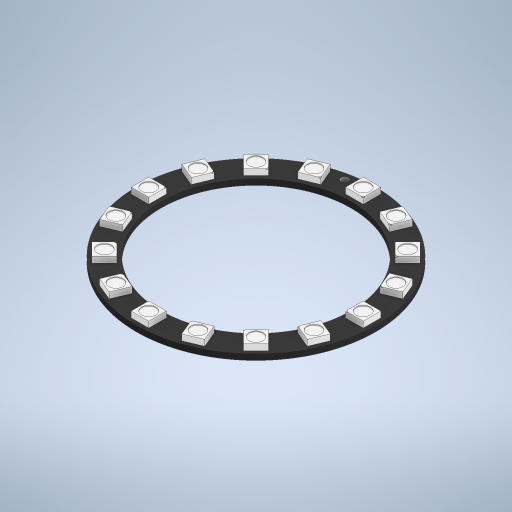
# Autodesk Inventor part: Neopixel circle
Saved by Autodesk Inventor 2023 (Build 270158000, 158)
## iProperties
Created: 2022-05-23
Part Number: Neopixel circle
Material: 일반
Document SubType Name: Modeling
Designer: user
Density: 1 g/cm^3
Appearance: 기본값
Author: user
Autodesk Inventor part; units mm, degrees
ref_plane "YZ Plane" through (0, 0, 0) normal (1, 0, 0) x (0, 1, 0)
ref_plane "XZ Plane" through (0, 0, 0) normal (0, 1, 0) x (-1, 0, 0)
ref_plane "XY Plane" through (0, 0, 0) normal (0, 0, 1) x (1, 0, 0)
sketch "스케치2" plane through (0, 0, 0) normal (0, 1, 0) x (-1, 0, 0)
  circle A0 centre (0, 0) radius 34
  circle A1 centre (0, 0) radius 27
  line L0 (33, 2.5) -> (28, 2.5)
  line L1 (28, 2.5) -> (28, -2.5)
  line L2 (28, -2.5) -> (33, -2.5)
  line L3 (33, -2.5) -> (33, 2.5)
  line L4 (33, 2.5) -> (28, -2.5) construction
  line L5 (28, 2.5) -> (33, -2.5) construction
  point P0 (30.5, 0)
  dimension "d0" = 68
  dimension "d1" = 54
  dimension "d2" = 5
  dimension "d3" = 5
  dimension "d4" = 33
  constraints: 12 end point, 2 centre point, 2 coincident, 2 midpoint, 2 parallel, 1 horizontal, 1 perpendicular
  measures "d0" diameter of A0
  measures "d1" diameter of A1
  measures "d2" distance of L2.end L1.end
  measures "d3" distance of L1.end L0.end
  measures "d4" distance from line of A0.centre L3
extrude "돌출1" add sketch "스케치2" against normal blind 1.7 contours A0 | L3 L2 L1 L0
extrude "돌출2" add sketch "스케치2" along normal blind 1.7 contours L3 L2 L1 L0
sketch "스케치3" plane through (0, 1.7, 0) normal (0, 1, 0) x (1, 0, 0)
  line L0 (-28, -2.5) -> (-28, 2.5) projected
  line L1 (-28, 2.5) -> (-33, 2.5) projected
  line L2 (-33, 2.5) -> (-33, -2.5) projected
  line L3 (-33, -2.5) -> (-28, -2.5) projected
  line L4 (-33, 2.5) -> (-33, -2.5) projected
  line L5 (-28, -2.5) -> (-28, 2.5) projected
  line L6 (-33, -2.5) -> (-28, 2.5)
  circle A0 centre (-30.5, 0) radius 2
  line L7 (-28, 2) -> (-28.5, 2.5)
  line L8 (-28, 2.5) -> (-33, 2.5) projected
  point P0 (0, 0)
  dimension "d9" = 4
  constraints: 4 end point, 2 point on line, 1 centre point, 1 midpoint
  measures "d9" diameter of A0
extrude "돌출3" cut sketch "스케치3" against normal blind 0.2 contours L7 L6 L0 | L6 L7 L1 | A0 L6 | L6 A0
pattern_circular "원형 패턴1" count 16 over 360 about axis through (0, 0, 0) along (0, -1, 0) of "돌출3", "돌출2"
sketch "스케치4" plane through (0, 0, 0) normal (0, 1, 0) x (1, 0, 0)
  line L0 (-14.9383, 29.5313) -> (-10.3189, 31.4447) projected
  line L1 (-2.5, 33) -> (-2.5, 28) projected
  line L2 (-8.4054, 26.8253) -> (-2.5, 28)
  line L3 (-5.4527, 27.4127) -> (-6.6331, 33.3467)
  circle A0 centre (0, 0) radius 34 projected
  circle A1 centre (-6.2539, 31.4407) radius 1
  line L4 (-6.6331, 33.3467) -> (-6.2429, 31.3851)
  circle A2 centre (0, 0) radius 32
  dimension "d15" = 2
  dimension "d16" = 2
  constraints: 6 end point, 2 coincident, 2 point on line, 1 centre point, 1 midpoint, 1 perpendicular, 5 other
  measures "d15" diameter of A1
  measures "d16" distance of L3.end L4.end
extrude "돌출4" cut sketch "스케치4" against normal blind 10 contours A2 L3 A1 | A1 L3 A2 | A2 L3 A1 | A1 L3 A2
